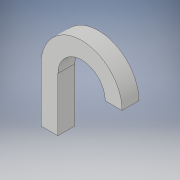
# Autodesk Inventor part: TelescopeHook
Saved by Autodesk Inventor 2018.3 (Build 223284000, 284)
## iProperties
Created: 2020-01-18
Part Number: TelescopeHook
Material: Generic
Document SubType Name: Modeling
Designer: Cooper
Density: 1 g/cm^3
Appearance: Default
Mass: 36.683 g
Surface Area: 97.4698 cm^2
Volume: 36.683 cm^3
Author: Cooper
Autodesk Inventor part; units mm, degrees
ref_plane "YZ Plane" through (0, 0, 0) normal (1, 0, 0) x (0, 1, 0)
ref_plane "XZ Plane" through (0, 0, 0) normal (0, 1, 0) x (-1, 0, 0)
ref_plane "XY Plane" through (0, 0, 0) normal (0, 0, 1) x (1, 0, 0)
sketch "Sketch1" plane through (0, 0, 0) normal (0, 0, 1) x (1, 0, 0)
  line L0 (0, 0) -> (0, 50.8)
  line L1 (-12.3149, 50.587) -> (-12.3149, 50.587)
  arc A0 (76.2, 50.8) -> (0, 50.8) centre (38.1, 50.8) ccw
  line L2 (0, 0) -> (15.875, 0)
  line L3 (15.875, 0) -> (15.875, 50.8)
  arc A1 (60.325, 50.8) -> (15.875, 50.8) centre (38.1, 50.8) ccw
  line L4 (76.2, 50.8) -> (60.325, 50.8)
  line L5 (8.5732, 88.9) -> (68.624, 88.9) construction
  dimension "d1" = 15.875
  dimension "d3" = 50.8
  dimension "d6" = 38.1
  constraints: 12 end point, 4 point on circle, 3 horizontal, 3 tangent, 2 centre point, 2 parallel, 1 coincident, 1 perpendicular, 1 vertical
  measures "d1" distance of L0.start L2.end
  measures "d3" distance of L0.start L0.end
  measures "d6" distance from line of L0.end L5
extrude "Extrusion1" add sketch "Sketch1" along normal blind 15.875
equation "\"d4\" = d1"
body "Solid1"
